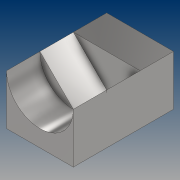
# Autodesk Inventor part: 38
Saved by Autodesk Inventor 2020.2 (Build 242310000, 310)
## iProperties
Created: 2020-09-17
Part Number: 38
Material: 鋼、碳鋼
Document SubType Name: Modeling
Designer: user
Density: 7.85 g/cm^3
Appearance: 半拋光
Mass: 403.754 g
Surface Area: 115.88 cm^2
Volume: 51.4336 cm^3
Author: user
Autodesk Inventor part; units mm, degrees
ref_plane "YZ Plane" through (0, 0, 0) normal (1, 0, 0) x (0, 1, 0)
ref_plane "XZ Plane" through (0, 0, 0) normal (0, 1, 0) x (-1, 0, 0)
ref_plane "XY Plane" through (0, 0, 0) normal (0, 0, 1) x (1, 0, 0)
sketch "草圖1" plane through (0, 0, 0) normal (0, 1, 0) x (-1, 0, 0)
  line L0 (20, 0) -> (-20, 0)
  line L1 (-20, 0) -> (-20, 60)
  line L2 (-20, 60) -> (20, 60)
  line L3 (20, 60) -> (20, 0)
  point P0 (0, 0)
  point P1 (0, 0)
  dimension "d0" = 40
  dimension "d1" = 60
  constraints: 8 end point, 2 parallel, 1 coincident, 1 horizontal, 1 midpoint, 1 perpendicular
  measures "d0" distance of L1.end L2.end
  measures "d1" distance of L0.end L1.end
extrude "擠出1" add sketch "草圖1" along normal blind 30
sketch "草圖2" plane through (-20, 0, 60) normal (0, 0, 1) x (1, 0, 0)
  line L0 (0, 0) -> (0, 30) projected
  line L1 (0, 30) -> (40, 30) projected
  line L2 (40, 30) -> (40, 0) projected
  line L3 (40, 0) -> (0, 0) projected
  line L4 (40, 30) -> (0, 30) projected
  arc A0 (0, 30) -> (40, 30) centre (20, 30) ccw
  point P0 (20, 0)
  constraints: 2 end point, 2 point on circle, 1 centre point, 1 midpoint
extrude "擠出2" cut sketch "草圖2" against normal blind 20 contours L1 A0
sketch "草圖3" plane through (-20, 0, 40) normal (0, 0, 1) x (1, 0, 0)
  arc A0 (0, 30) -> (40, 30) centre (20, 30) ccw projected
  line L0 (0, 30) -> (40, 30) projected
  line L1 (0, 0) -> (0, 30) projected
  line L2 (40, 0) -> (0, 0) projected
  line L3 (40, 30) -> (40, 0) projected
  line L4 (0, 0) -> (0, 30) projected
  line L5 (0, 30) -> (20, 10)
  line L6 (40, 30) -> (0, 30) projected
  line L7 (20, 10) -> (40, 30)
  line L8 (40, 30) -> (0, 30)
  point P0 (20, 0)
  constraints: 6 end point, 2 perpendicular, 1 point on circle
extrude "擠出3" cut sketch "草圖3" against normal blind 20 contours L0 L7 L5
